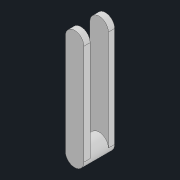
# Autodesk Inventor part: link2
Saved by Autodesk Inventor 2021 (Build 250183000, 183)
## iProperties
Created: 2021-07-10
Part Number: link2
Material: 一般
Document SubType Name: Modeling
Designer: yuta0
Density: 1 g/cm^3
Appearance: 既定
Author: yuta0
Autodesk Inventor part; units mm, degrees
ref_plane "YZ Plane" through (0, 0, 0) normal (1, 0, 0) x (0, 1, 0)
ref_plane "XZ Plane" through (0, 0, 0) normal (0, 1, 0) x (-1, 0, 0)
ref_plane "XY Plane" through (0, 0, 0) normal (0, 0, 1) x (1, 0, 0)
sketch "スケッチ1" plane through (0, 0, 0) normal (0, 0, 1) x (1, 0, 0)
  circle A0 centre (0, 0) radius 40.5
  circle A1 centre (0, 440) radius 40.5
  line L0 (-40.5, 440) -> (-40.5, 0)
  line L1 (40.5, 0) -> (40.5, 440)
  dimension "d0" = 81
  dimension "d1" = 81
  dimension "d2" = 440
  constraints: 4 end point, 4 point on circle, 4 tangent, 2 centre point, 1 coincident, 1 vertical alignment
  measures "d0" diameter of A0
  measures "d1" diameter of A1
  measures "d2" distance of A0.centre A1.centre
extrude "押し出し1" add sketch "スケッチ1" along normal mid plane 135
sketch "スケッチ2" plane through (0, 0, 0) normal (0, 0, 1) x (1, 0, 0)
  arc A0 (-40.5, 0) -> (40.5, 0) centre (0, 0) ccw projected
  line L0 (-40.5, 0) -> (-40.5, 440) projected
  arc A1 (40.5, 440) -> (-40.5, 440) centre (0, 440) ccw projected
  line L1 (40.5, 440) -> (40.5, 0) projected
  arc A2 (-40.5, 0) -> (40.5, 0) centre (0, 0) ccw projected
  line L2 (-40.5, 0) -> (-40.5, 440) projected
  arc A3 (40.5, 440) -> (-40.5, 440) centre (0, 440) ccw projected
  line L3 (40.5, 440) -> (40.5, 0) projected
extrude "押し出し2" cut sketch "スケッチ2" along normal mid plane 80
sketch "スケッチ3" plane through (0, 0, -40) normal (0, 0, 1) x (1, 0, 0)
  circle A0 centre (0, 0) radius 40.5
  point P0 (40.5, 0)
  constraints: 1 coincident, 1 horizontal alignment, 2 other
extrude "押し出し3" add sketch "スケッチ3" along normal up to surface (80 mm away)
